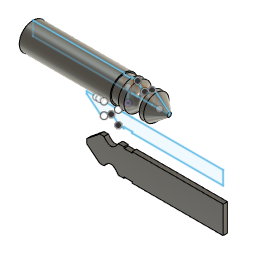
2022_09_03_MidiJack v3 (Autodesk Fusion 360 design; units mm, degrees)
Autodesk Fusion 360 part; units mm, degrees
sketch "Sketch1" plane through (0, 0, 0) normal (1, 0, 0) x (0, 1, 0)
  circle A0 centre (0, 0) radius 3.15
  circle A1 centre (0, 0) radius 1.85
  circle A2 centre (0, 0) radius 0.75
  circle A3 centre (0, 0) radius 2.9
  dimension "d1" = 6.3
  dimension "d4" = 3.7
  dimension "d5" = 1.5
  dimension "d6" = 5.8
  constraint coincident A0.centre A1.centre
  constraint concentric A1 A2
  measures "d1" diameter of A0
  measures "d4" diameter of A1
  measures "d5" diameter of A2
  measures "d6" diameter of A3
extrude "Extrude2" add sketch "Sketch1" along normal blind 1.4 contours A1 | A2 | A3 makes body 1
extrude "Extrude1" add sketch "Sketch1" along normal blind 31 separate body contours A0 | A1 | A2 | A3 makes body 2
sketch "Sketch2" plane through (0, 0, 0) normal (0, 1, 0) x (1, 0, 0)
sketch "JackTipMeasureByHand" plane through (0, 0, 0) normal (0, 1, 0) x (1, 0, 0)
  line L0 (0, 0) -> (0, -3.15)
  line L1 (2.2338, -5.1672) -> (5.5338, -5.1672)
  line L2 (5.5338, -5.1672) -> (5.5338, -2.4006)
  line L3 (5.5338, -2.4006) -> (2.2338, -2.4006)
  line L4 (2.2338, -2.4006) -> (2.2338, -5.1672)
  line L5 (5.5338, -2.4006) -> (6.5338, -2.4006)
  line L6 (6.5338, -2.4006) -> (6.5338, -5.3256)
  line L7 (6.5338, -5.3256) -> (5.5338, -5.3256)
  line L8 (5.5338, -5.3256) -> (5.5338, -2.4006)
  line L9 (6.5338, -2.4006) -> (9.5338, -2.4006)
  line L10 (9.5338, -2.4006) -> (9.5338, -2.9006)
  line L11 (9.5338, -2.9006) -> (6.5338, -2.9006)
  line L12 (6.5338, -2.9006) -> (6.5338, -2.4006)
  line L13 (2.2338, -2.4006) -> (0.9338, -2.4006)
  line L14 (0.9338, -2.4006) -> (2.2338, -2.4006)
  line L15 (2.2338, -2.4006) -> (2.2338, -5.5506)
  line L16 (2.2338, -5.5506) -> (0.9338, -5.5506)
  line L17 (0.9338, -5.5506) -> (0.9338, -2.4006)
  line L18 (3.8838, -2.4006) -> (3.8838, -4.2006)
  spline S0 degree 5 poles (2.2338, -5.5506) (2.2985, -5.4527) (2.428, -5.2649) (2.6225, -5.0076) (2.8826, -4.7141) (3.2089, -4.4353) (3.5366, -4.2528) (3.8659, -4.1745) (4.1966, -4.2053) (4.5289, -4.3414) (4.8625, -4.5749) (5.1304, -4.8334) (5.3319, -5.0651) (5.4665, -5.236) (5.5338, -5.3256) knots 0 0 0 0 0 0 0.1 0.2 0.3 0.4 0.5 0.6 0.7 0.8 0.9 1 1 1 1 1 1
  line L19 (6.5338, -5.3256) -> (9.5338, -2.9006)
  line L20 (5.5338, -2.4006) -> (7.2338, -2.4006)
  line L21 (5.5338, -2.4006) -> (2.2338, -2.4006)
  line L22 (2.2338, -2.4006) -> (0.9338, -2.4006)
  line L23 (0.9338, -5.5506) -> (0.9338, -2.4006)
  line L24 (2.2338, -5.5506) -> (0.9338, -5.5506)
  spline S1 degree 5 poles (2.2338, -5.5506) (2.2985, -5.4527) (2.428, -5.2649) (2.6225, -5.0076) (2.8826, -4.7141) (3.2089, -4.4353) (3.5366, -4.2528) (3.8659, -4.1745) (4.1966, -4.2053) (4.5289, -4.3414) (4.8625, -4.5749) (5.1304, -4.8334) (5.3319, -5.0651) (5.4665, -5.236) (5.5338, -5.3256) knots 0 0 0 0 0 0 0.1 0.2 0.3 0.4 0.5 0.6 0.7 0.8 0.9 1 1 1 1 1 1
  line L25 (0.9338, -2.4006) -> (-0.9662, -2.4006)
  line L26 (-0.9662, -2.4006) -> (-0.9662, -5.2602)
  line L27 (-0.9662, -5.2602) -> (0.9338, -5.2602)
  line L28 (0.9338, -5.2602) -> (0.9338, -2.4006)
  line L29 (-0.9662, -2.4006) -> (-21.9662, -2.4006)
  line L30 (-21.9662, -2.4006) -> (-21.9662, -5.5506)
  line L31 (-21.9662, -5.5506) -> (-0.9662, -5.5506)
  line L32 (-0.9662, -5.5506) -> (-0.9662, -2.4006)
  line L33 (-0.9662, -5.2602) -> (-0.9662, -5.5506)
  line L34 (0.9338, -5.2602) -> (0.9338, -5.5506)
  point P0 (3.8838, -4.2006)
  dimension "d9" = 3.15
  dimension "d11" = 3.3
  dimension "d12" = 1
  dimension "d13" = 2.925
  dimension "d14" = 3
  dimension "d15" = 0.5
  dimension "d16" = 2.7666
  dimension "d18" = 1.3
  dimension "d19" = 1.3
  dimension "d20" = 3.15
  dimension "d21" = 1.8
  dimension "d22" = 1.7
  dimension "d23" = 2.925
  dimension "d25" = 1.3
  dimension "d26" = 3.15
  dimension "d27" = 1.9
  dimension "d28" = 21
  dimension "d29" = 3.15
  constraint coincident L0.start origin
  constraint horizontal L1
  constraint vertical L2
  constraint horizontal L3
  constraint horizontal L5
  constraint vertical L6
  constraint horizontal L7
  constraint vertical L8
  constraint horizontal L9
  constraint vertical L10
  constraint horizontal L11
  constraint vertical L12
  constraint perpendicular L4 L13
  constraint horizontal L14
  constraint vertical L15
  constraint horizontal L16
  constraint vertical L17
  constraint midpoint L3 L18.start
  constraint perpendicular L3 L18
  constraint horizontal L21
  constraint horizontal L20
  constraint horizontal L24
  constraint vertical L23
  constraint horizontal L25
  constraint vertical L26
  constraint horizontal L27
  constraint vertical L28
  constraint horizontal L29
  constraint vertical L30
  constraint horizontal L31
  constraint vertical L32
  constraint perpendicular L31 L33
  constraint perpendicular L24 L34
  measures "d9" distance of L0.start L0.end
  measures "d11" distance of L1.start L1.end
  measures "d12" distance of L2.end L5.end
  measures "d13" distance of L2.end L7.end
  measures "d14" distance of L5.end L9.end
  measures "d15" distance of L5.end L11.end
  measures "d16" distance of L1.start L3.end
  measures "d18" distance of L3.end L13.end
  measures "d19" distance of L13.end L3.end
  measures "d20" distance of L13.end L16.end
  measures "d21" distance of L18.start P0
  measures "d22" distance of L20.end L2.end
  measures "d23" distance of L7.end L2.end
  measures "d25" distance of L3.end L13.end
  measures "d26" distance of L16.end L13.end
  measures "d27" distance of L13.end L25.end
  measures "d28" distance of L25.end L29.end
  measures "d29" distance of L25.end L31.end
revolve "Revolve2" add sketch "JackTipMeasureByHand" angle 360 about axis through (-0.9662, 0, 2.4006) along (-1, 0, 0) separate body contours L1 L3 L4 L15 L18 S0 L21 S1 | L4 L13 L14 L15 L16 L17 L22 L23 L24 L28 L34 | L1 L15 S0 S1 | L1 L2 L3 L8 L18 S0 L21 S1 | L1 L8 S0 S1 | L17 L23 L25 L26 L27 L28 L32 | L2 L5 L6 L7 L8 L12 L20 | L6 L11 L19 | L6 L9 L10 L11 L12 L20 | L26 L29 L30 L31 L32 L33 makes body 3
sketch "JackSVG" plane through (0, 0, 0) normal (0, 1, 0) x (-1, 0, 0)
  line L0 (0.9338, -2.4006) -> (-0.9662, -2.4006)
  line L1 (-0.9662, -2.4006) -> (-21.9662, -2.4006)
  line L2 (-21.9662, -2.4006) -> (-21.9662, -5.5506)
  line L3 (-21.9662, -5.5506) -> (-0.9662, -5.5506)
  line L4 (-0.9662, -5.2602) -> (-0.9662, -5.5506)
  line L5 (-0.9662, -5.2602) -> (0.9338, -5.2602)
  line L6 (0.9338, -5.2602) -> (0.9338, -5.5506)
  line L7 (2.2338, -5.5506) -> (0.9338, -5.5506)
  spline S0 degree 5 poles (2.2338, -5.5506) (2.2985, -5.4527) (2.428, -5.2649) (2.6225, -5.0076) (2.8826, -4.7141) (3.2089, -4.4353) (3.5366, -4.2528) (3.8659, -4.1745) (4.1966, -4.2053) (4.5289, -4.3414) (4.8625, -4.5749) (5.1304, -4.8334) (5.3319, -5.0651) (5.4665, -5.236) (5.5338, -5.3256) knots 0 0 0 0 0 0 0.1 0.2 0.3 0.4 0.5 0.6 0.7 0.8 0.9 1 1 1 1 1 1
  line L8 (0.9338, -2.4006) -> (2.2338, -2.4006)
  line L9 (5.5338, -2.4006) -> (2.2338, -2.4006)
  line L10 (5.5338, -2.4006) -> (7.2338, -2.4006)
  line L11 (6.5338, -2.4006) -> (9.5338, -2.4006)
  line L12 (6.5338, -5.3256) -> (9.5338, -2.9006)
  line L13 (6.5338, -5.3256) -> (5.5338, -5.3256)
  line L14 (9.5338, -2.4006) -> (9.5338, -2.9006)
  point P0 (3.8838, -4.2006)
  dimension "d42" = 1
  dimension "d43" = 2.925
  dimension "d44" = 3
  dimension "d45" = 1.3
  dimension "d46" = 1.3
  dimension "d47" = 1.7
  dimension "d48" = 2.925
  dimension "d49" = 1.9
  dimension "d50" = 21
  dimension "d51" = 3.15
  constraint horizontal L9
  constraint horizontal L13
  constraint horizontal L11
  constraint vertical L14
  constraint horizontal L8
  constraint horizontal L10
  constraint horizontal L7
  constraint horizontal L0
  constraint horizontal L5
  constraint horizontal L1
  constraint vertical L2
  constraint horizontal L3
  constraint perpendicular L3 L4
  constraint perpendicular L6 L7
  measures "d42" distance of L11.start L9.start
  measures "d43" distance of S0.end L9.start
  measures "d44" distance of L11.end L11.start
  measures "d45" distance of L8.end L0.start
  measures "d46" distance of L8.end L0.start
  measures "d47" distance of L9.start L10.end
  measures "d48" distance of L9.start S0.end
  measures "d49" distance of L0.end L0.start
  measures "d50" distance of L0.end L1.end
  measures "d51" distance of L0.end L3.end
extrude "Extrude3" add sketch "JackSVG" along normal blind 1 separate body makes body 4
copy_body "CopyPasteBodies1" bodies 4 makes body 5
move_body "Move1" bodies 5 to x (1, 0, 0) y (0, -1, 0) z (0, 0, -1) at (0, 0, -4.8013)
move_body "Move2" bodies 5 to x (1, 0, 0) y (0, 1, 0) z (0, 0, 1) at (0, 1, 0)
combine "Combine1" operation add target body 5 tool bodies 4
move_body "Move3" bodies 5 to x (1, 0, 0) y (0, 1, 0) z (0, 0, 1) at (0, 0, -10)
hidden bodies 1 2
equation "d9 = ( 6.3 / 2 ) * 1 mm"
equation "d13 = 5.85 mm / 2"
equation "d15 = 1 mm / 2"
equation "d16 = 5.533238 mm / 2"
equation "d21 = ( 3.6 / 2 ) * 1 mm"
equation "d23 = 5.85 mm / 2"
equation "d29 = ( 6.3 / 2 ) * 1 mm"
equation "d43 = 5.85 mm / 2"
equation "d48 = 5.85 mm / 2"
equation "d51 = ( 6.3 / 2 ) * 1 mm"
